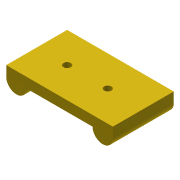
# Autodesk Inventor part: locator
Saved by Autodesk Inventor 2022 Beta2 (Build 260130000, 130) ContinuousBuild 0
## iProperties
Shininess: 64.0
Length Units: 11272
Angle Units: 11279
Time Units: 11290
Mass Units: 11286
Length Display Precision: 3
Angle Display Precision: 2
Created: 2002-02-11
Part Number: locator
Document SubType Name: Modeling
Designer: Administrator
Density: 1 g/cm^3
Material: Generic
Appearance: Glossy - Gold
Density: 0.0
Volumn: 0.0
Area: 0.0
PropertySet Name: Model Information
Control State: 0
Master: False
Checked Out: False
Author: Administrator
Autodesk Inventor part; units mm, degrees
ref_plane "YZ Plane" through (0, 0, 0) normal (1, 0, 0) x (0, 1, 0)
ref_plane "XZ Plane" through (0, 0, 0) normal (0, 1, 0) x (-1, 0, 0)
ref_plane "XY Plane" through (0, 0, 0) normal (0, 0, 1) x (1, 0, 0)
sketch "Sketch1" plane through (0, 0, 0) normal (0, 0, 1) x (1, 0, 0)
  line L0 (-48.1538, -4.158) -> (-48.1538, 2.192)
  line L1 (-48.1538, 2.192) -> (18.5212, 2.192)
  line L2 (18.5212, 2.192) -> (18.5212, -4.158)
  arc A0 (5.8212, -4.158) -> (18.5212, -4.158) centre (12.1712, -4.158) ccw
  line L3 (5.8212, -4.158) -> (-35.4538, -4.158)
  arc A1 (-48.1538, -4.158) -> (-35.4538, -4.158) centre (-41.8038, -4.158) ccw
  dimension "d0" = 6.35
  dimension "d1" = 6.35
  dimension "d2" = 66.675
  constraints: 8 end point, 4 point on circle, 2 centre point, 2 horizontal alignment, 2 parallel, 2 tangent, 1 equal radius, 1 perpendicular, 1 point on line, 1 vertical
  measures "d0" radius of A1
  measures "d1" distance of L1.end L2.end
  measures "d2" distance of L0.end L1.end
extrude "Extrusion1" add sketch "Sketch1" along normal blind 38.1
sketch "Sketch2" plane through (-48.1538, 2.192, 0) normal (0, 1, 0) x (1, 0, 0)
  line L0 (0, 0) -> (0, -38.1) projected
  line L1 (19.05, -19.05) -> (44.45, -19.05)
  point P0 (66.675, 0)
  dimension "d5" = 22.225
  dimension "d6" = 25.4
  dimension "d7" = 19.05
  constraints: 2 end point, 1 perpendicular
  measures "d5" horizontal distance of point (66.675, 0) L1.end
  measures "d6" distance of L1.start L1.end
  measures "d7" vertical distance of point (66.675, 0) L1.end
hole "Hole1" at (-3.7038, 2.192, 19.05) at (-29.1038, 2.192, 19.05) direction (0, -1, 0) diameter 4.572 end through all
body "Solid1"
